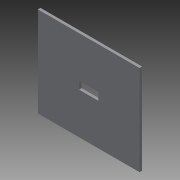
# Autodesk Inventor part: Surface Switch Cutout
Saved by Autodesk Inventor 2015 (Build 190159000, 159)
## iProperties
Created: 2015-02-05
Part Number: Surface Switch Cutout
Material: Generic
Document SubType Name: Modeling
Designer: robotics
Density: 1 g/cm^3
Appearance: Default
Author: robotics
Autodesk Inventor part; units mm, degrees
ref_plane "YZ Plane" through (0, 0, 0) normal (1, 0, 0) x (0, 1, 0)
ref_plane "XZ Plane" through (0, 0, 0) normal (0, 1, 0) x (-1, 0, 0)
ref_plane "XY Plane" through (0, 0, 0) normal (0, 0, 1) x (1, 0, 0)
sketch "Sketch1" plane through (0, 0, 0) normal (0, 0, 1) x (1, 0, 0)
  line L0 (-14.8528, 1.9795) -> (12.8586, 1.9795) construction
  line L1 (12.8586, 1.9795) -> (12.8586, -13.7685) construction
  line L2 (12.8586, -13.7685) -> (-14.8528, -13.7685) construction
  line L3 (-14.8528, -13.7685) -> (-14.8528, 1.9795) construction
  line L4 (5.9975, 1.9795) -> (8.6518, 1.9795) construction
  line L5 (8.6518, 1.9795) -> (8.6518, 4.3671) construction
  line L6 (8.6518, 4.3671) -> (5.9975, 4.3671) construction
  line L7 (5.9975, 4.3671) -> (5.9975, 1.9795) construction
  line L8 (-32.4421, 11.5045) -> (30.2817, 11.5045) construction
  line L9 (-32.4421, 8.3295) -> (29.9988, 8.3295) construction
  line L10 (-13.9321, 13.8921) -> (17.834, 13.8921) construction
  line L11 (-1.8734, -10.8674) -> (-1.8734, -21.0274) construction
  line L12 (-2.2544, -23.9285) -> (-2.2544, -13.7685) construction
  line L13 (-14.8528, -9.4505) -> (-21.958, -9.4505) construction
  line L14 (-21.958, -9.8315) -> (-14.0038, -9.8315) construction
  line L15 (-14.8528, 1.9795) -> (12.6787, 5.1322) construction
  arc A0 (9.1943, 9.241) -> (-14.8528, 1.9795) centre (-1.1526, 0.0577) ccw construction
  circle A1 centre (-10.8004, 5.3198) radius 0.889 construction
  line L16 (-13.0354, 11.5045) -> (-13.0354, 8.3295) construction
  line L17 (10.7302, 11.5045) -> (10.7302, 8.3295) construction
  line L18 (-12.2416, 8.3295) -> (-12.2416, 11.5045) construction
  line L19 (9.9365, 8.3295) -> (9.9365, 11.5045) construction
  line L20 (13.1115, 8.3295) -> (11.9301, 8.1942) construction
  line L21 (11.9301, 8.1942) -> (12.3229, 8.2392) construction
  line L22 (13.377, 6.0111) -> (13.2018, 7.5409) construction
  line L23 (-13.2979, 6.6819) -> (-11.5809, 5.7454) construction
  line L24 (-10.4753, 2.4807) -> (-10.6993, 4.4365) construction
  arc A2 (9.1943, 9.241) -> (11.9301, 8.1942) centre (11.5689, 11.3486) ccw construction
  arc A3 (13.2018, 7.5409) -> (12.3229, 8.2392) centre (12.4132, 7.4506) ccw construction
  arc A4 (12.6787, 5.1322) -> (13.377, 6.0111) centre (12.5884, 5.9208) ccw construction
  circle A5 centre (-11.9953, -0.878) radius 1.5875 construction
  line L25 (-13.5828, 0.7095) -> (-5.6621, 0.7095) construction
  line L26 (-13.5828, -2.3385) -> (-13.5828, 0.7095) construction
  circle A6 centre (10.0011, -10.911) radius 1.5875 construction
  line L27 (11.5886, -9.3235) -> (11.5886, -12.4985) construction
  line L28 (11.5886, -12.4985) -> (4.7585, -12.4985) construction
  line L29 (-13.0354, 11.5045) -> (10.7302, 11.5045)
  line L30 (10.7302, 11.5045) -> (10.7302, 21.0295)
  line L31 (10.7302, 21.0295) -> (-13.0354, 21.0295)
  line L32 (-13.0354, 21.0295) -> (-13.0354, 11.5045)
  line L33 (-63.8354, 71.8295) -> (61.5302, 71.8295)
  line L34 (61.5302, 71.8295) -> (61.5302, -39.2955)
  line L35 (61.5302, -39.2955) -> (-63.8354, -39.2955)
  line L36 (-63.8354, -39.2955) -> (-63.8354, 71.8295)
  point P0 (0, 0)
  dimension "d0" = 27.7114
  dimension "d1" = 15.748
  dimension "d2" = 2.6543
  dimension "buttonHeight" = 2.3876
  dimension "d4" = 3.175
  dimension "d5" = 2.3876
  dimension "buttonInset" = 4.2068
  dimension "d10" = 14.732
  dimension "d11" = 0.381
  dimension "d12" = 10.16
  dimension "d14" = 11.43
  dimension "d15" = 0.381
  dimension "d16" = 6.35
  dimension "nail" = 1.778
  dimension "clearance" = 0.7937
  dimension "d32" = 0.7937
  dimension "cutOutLength" = 23.7656
  dimension "d34" = 2.3813
  dimension "d35" = 1.9558
  dimension "d36" = 1.9558
  dimension "d37" = 3.175
  dimension "d38" = 0.7937
  dimension "holeDistanceFromSurface" = 3.0097
  dimension "holeDistanceFromEnd" = 4.0524
  dimension "d52" = 3.175
  dimension "d53" = 1.27
  dimension "d54" = 1.27
  dimension "d55" = 3.175
  dimension "d56" = 1.27
  dimension "d57" = 1.27
  dimension "d60" = 9.525
  dimension "d63" = 50.8
  dimension "d64" = 50.8
  dimension "d65" = 50.8
  dimension "d66" = 50.8
  constraints: 74 end point, 17 point on line, 14 point on circle, 11 parallel, 11 tangent, 10 perpendicular, 9 horizontal, 7 centre point, 3 line through centre, 2 collinear, 1 equal length, 1 equal radius
  measures "d0" distance of L1.end L2.end
  measures "d1" distance of L0.end L1.end
  measures "d2" distance of L5.end L6.end
  measures "buttonHeight" distance of L4.end L5.end
  measures "d4" distance between parallel lines of L9 L8
  measures "d5" distance between parallel lines of L8 L10
  measures "buttonInset" distance between parallel lines of L1 L5
  measures "d10" distance between parallel lines of L1 L11
  measures "d11" distance between parallel lines of L11 L12
  measures "d12" distance of L12.start L12.end
  measures "d14" distance between parallel lines of L13 L0
  measures "d15" distance between parallel lines of L14 L13
  measures "d16" distance between parallel lines of L0 L9
  measures "nail" diameter of A1
  measures "clearance" distance between parallel lines of L16 L18
  measures "d32" distance between parallel lines of L17 L19
  measures "cutOutLength" distance between parallel lines of L17 L16
  measures "d34" distance from line of L17 L20.start
  measures "d35" distance of L23.start L23.end
  measures "d36" vertical distance of L24.start L24.end
  measures "d37" radius of A2
  measures "d38" radius of A3
  measures "holeDistanceFromSurface" distance from line of L9 A1.centre
  measures "holeDistanceFromEnd" distance from line of L3 A1.centre
  measures "d52" diameter of A5
  measures "d53" distance between parallel lines of L0 L25
  measures "d54" distance from line of L3 L26.start
  measures "d55" diameter of A6
  measures "d56" distance between parallel lines of L2 L28
  measures "d57" distance between parallel lines of L1 L27
  measures "d60" distance of L29.end L30.end
  measures "d63" distance between parallel lines of L33 L31
  measures "d64" distance between parallel lines of L34 L30
  measures "d65" distance between parallel lines of L35 L29
  measures "d66" distance between parallel lines of L36 L32
extrude "Extrusion7" add sketch "Sketch1" along normal blind 3.175
equation "\"d5\" = buttonHeight"
equation "\"d32\" = clearance"
body "Solid4"
